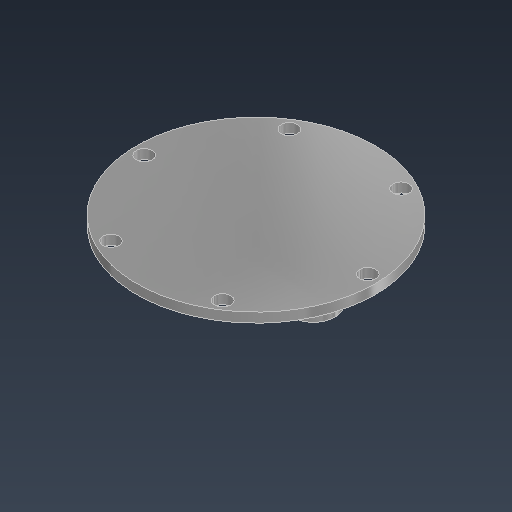
# Autodesk Inventor part: P019-Chapeau_tete_chambre
Saved by Autodesk Inventor 2021.3 (Build 253353000, 353)
## iProperties
Created: 2022-05-29
Part Number: P019-Chapeau_tete_chambre
Material: Aluminium
Document SubType Name: Modeling
Designer: Rémi Heredero
Density: 2.7 g/cm^3
Appearance: Aluminum - Dark
Author: Rémi Heredero
Autodesk Inventor part; units mm, degrees
ref_plane "YZ Plane" through (0, 0, 0) normal (1, 0, 0) x (0, 1, 0)
ref_plane "XZ Plane" through (0, 0, 0) normal (0, 1, 0) x (-1, 0, 0)
ref_plane "XY Plane" through (0, 0, 0) normal (0, 0, 1) x (1, 0, 0)
sketch "Sketch2" plane through (0, 0, 0) normal (0, 0, 1) x (1, 0, 0)
  circle A0 centre (0, 0) radius 25
  dimension "d0" = 50
  constraints: 1 centre point, 1 coincident
  measures "d0" diameter of A0
extrude "Extrusion1" add sketch "Sketch2" along normal blind 2
sketch "Sketch3" plane through (0, 0, 2) normal (0, 0, 1) x (1, 0, 0)
  circle A0 centre (-12.0283, 19.015) radius 1.2295 construction
  circle A1 centre (-10.4534, -19.9243) radius 1.2295 construction
  circle A2 centre (22.4816, 0.9093) radius 1.2295 construction
  circle A3 centre (12.0283, -19.015) radius 1.2295 construction
  circle A4 centre (-22.4816, -0.9093) radius 1.2295 construction
  circle A5 centre (10.4534, 19.9243) radius 1.2295 construction
  circle A6 centre (0, 0) radius 25 construction
  circle A7 centre (0, 0) radius 20 projected
  point P0 (0, 0)
hole "Hole1" at (22.4816, 0.9093, 2) at (12.0283, -19.015, 2) at (-10.4534, -19.9243, 2) at (-22.4816, -0.9093, 2) at (-12.0283, 19.015, 2) at (10.4534, 19.9243, 2) direction (0, 0, -1) diameter 3.4 end through all clearance for "Countersunk Flat Head Screw ISO 2009/7046" size "M3" standard "ISO"
sketch "Sketch4" plane through (0, 0, 0) normal (0, 0, -1) x (-1, 0, 0)
  circle A0 centre (-7.3947, 4.6777) radius 6 construction
  circle A1 centre (-7.3947, 4.6777) radius 4 construction
  circle A2 centre (-7.3947, 4.6777) radius 2.5
  circle A3 centre (-7.3947, 4.6777) radius 4.5
  point P0 (0, 0)
  dimension "d10" = 5
  dimension "d11" = 2
  constraints: 2 centre point, 2 coincident
  measures "d10" diameter of A2
  measures "d11" radial gap between concentric circles of A3 A2
extrude "Extrusion2" add sketch "Sketch4" along normal blind 13
body "Solid1"
